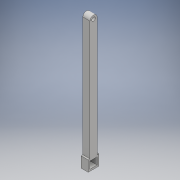
# Autodesk Inventor part: long extention
Saved by Autodesk Inventor 2018 (Build 220112000, 112)
## iProperties
Created: 2018-01-21
Part Number: long extention
Material: Generic
Document SubType Name: Modeling
Designer: omara
Density: 1 g/cm^3
Appearance: Default
Author: omara
Autodesk Inventor part; units mm, degrees
ref_plane "YZ Plane" through (0, 0, 0) normal (1, 0, 0) x (0, 1, 0)
ref_plane "XZ Plane" through (0, 0, 0) normal (0, 1, 0) x (-1, 0, 0)
ref_plane "XY Plane" through (0, 0, 0) normal (0, 0, 1) x (1, 0, 0)
sketch "Sketch1" plane through (0, 0, 0) normal (1, 0, 0) x (0, 1, 0)
  arc A0 (0, 266.1728) -> (-40, 266.1728) centre (-20, 266.1728) ccw
  circle A1 centre (-20, 266.1728) radius 10
  line L0 (0, 266.1728) -> (-10, 266.1728)
  line L1 (-0.0023, -412.6691) -> (-40.0023, -412.6691)
  line L2 (-40.0023, -412.6691) -> (-40.0023, -452.6691)
  line L3 (-40.0023, -452.6691) -> (-0.0023, -452.6691)
  line L4 (-0.0023, -452.6691) -> (-0.0023, -412.6691)
  line L5 (-50, -462.6691) -> (10, -462.6691)
  line L6 (10, -462.6691) -> (10, -402.6691)
  line L7 (10, -402.6691) -> (-50, -402.6691)
  line L8 (-50, -402.6691) -> (-50, -462.6691)
  line L9 (-40, 266.1728) -> (-40, -402.6691)
  line L10 (0, -402.6691) -> (0, 266.1728)
  point P0 (0, 0)
  dimension "d5" = 20
  dimension "d4" = 40
  dimension "d6" = 40
  dimension "d7" = 40
  dimension "d8" = 60
  dimension "d9" = 60
  dimension "d11" = 10
  dimension "d13" = 20
  constraints: 22 end point, 5 parallel, 3 horizontal, 3 perpendicular, 2 point on circle, 2 point on line, 1 centre point, 1 coincident, 1 horizontal alignment, 2 other
  measures "d4" diameter of A0
  measures "d6" distance of L3.end L2.end
  measures "d7" distance of L1.end L2.end
  measures "d8" distance of L7.end L6.end
  measures "d9" distance of L5.end L6.end
  measures "d11" distance between parallel lines of L1 L7
  measures "d13" radius of A0
extrude "Extrusion1" add sketch "Sketch1" along normal blind 40
body "Solid1"
